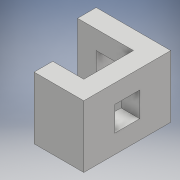
# Autodesk Inventor part: P3-4
Saved by Autodesk Inventor 2017 (Build 210142000, 142)
## iProperties
Created: 2017-02-10
Part Number: P3-4
Material: Generic
Document SubType Name: Modeling
Designer: Schaffel
Density: 1 g/cm^3
Appearance: Default
Author: Schaffel
Autodesk Inventor part; units mm, degrees
ref_plane "YZ Plane" through (0, 0, 0) normal (1, 0, 0) x (0, 1, 0)
ref_plane "XZ Plane" through (0, 0, 0) normal (0, 1, 0) x (-1, 0, 0)
ref_plane "XY Plane" through (0, 0, 0) normal (0, 0, 1) x (1, 0, 0)
sketch "Sketch1" plane through (0, 0, 0) normal (0, 0, 1) x (1, 0, 0)
  line L0 (20, 0) -> (60, 0)
  line L1 (60, 0) -> (60, 70)
  line L2 (60, 70) -> (0, 70)
  line L3 (0, 70) -> (0, 55)
  line L4 (0, 55) -> (45, 55)
  line L5 (45, 55) -> (45, 15)
  line L6 (45, 15) -> (20, 15)
  line L7 (20, 15) -> (20, 0)
  point P0 (0, 0)
  dimension "d0" = 40
  dimension "d1" = 70
  constraints: 16 end point, 6 perpendicular, 1 horizontal, 1 parallel
  measures "d0" distance of L0.start L0.end
  measures "d1" distance of L0.end L1.end
extrude "Extrusion1" add sketch "Sketch1" along normal blind 50
sketch "Sketch2" plane through (0, 70, 0) normal (0, 1, 0) x (1, 0, 0)
  line L0 (15, -15) -> (15, -35)
  line L1 (15, -35) -> (30, -35)
  line L2 (30, -35) -> (30, -15)
  line L3 (30, -15) -> (15, -15)
  point P0 (0, 0)
  constraints: 8 end point, 3 perpendicular, 1 vertical
extrude "Extrusion2" cut sketch "Sketch2" against normal blind 15
sketch "Sketch3" plane through (60, 0, 0) normal (1, 0, 0) x (0, 0, -1)
  line L0 (-15, 25) -> (-35, 25)
  line L1 (-35, 25) -> (-35, 45)
  line L2 (-35, 45) -> (-15, 45)
  line L3 (-15, 45) -> (-15, 25)
  point P0 (0, 0)
  constraints: 8 end point, 3 perpendicular, 1 horizontal
extrude "Extrusion3" cut sketch "Sketch3" against normal blind 15
body "Solid1"
